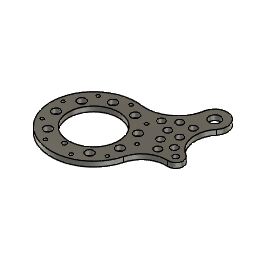
电机支架面板2 v8 (Autodesk Fusion 360 design; units mm, degrees)
Autodesk Fusion 360 part; units mm, degrees
sketch "草图1" plane through (0, 0, 0) normal (0, 0, 1) x (1, 0, 0)
  circle A0 centre (0, 0) radius 25
  circle A1 centre (0, 0) radius 37.5 construction
  circle A2 centre (0, 0) radius 42.5
  line L0 (0, 0) -> (0, 56.853) construction
  circle A3 centre (0, 37.5) radius 1.65
  circle A4 centre (-24.1045, 28.7267) radius 1.65
  circle A5 centre (-36.9303, 6.5118) radius 1.65
  circle A6 centre (-32.476, -18.75) radius 1.65
  circle A7 centre (-12.8258, -35.2385) radius 1.65
  circle A8 centre (12.8258, -35.2385) radius 1.65
  circle A9 centre (32.476, -18.75) radius 1.65
  circle A10 centre (36.9303, 6.5118) radius 1.65
  circle A11 centre (24.1045, 28.7267) radius 1.65
  line L1 (0, 0) -> (0, -49) construction
  circle A12 centre (0, -29) radius 2.2361
  dimension "d1" = 50
  dimension "d2" = 75
  dimension "d3" = 85
  dimension "d4" = 3.3
  dimension "d6" = 360
  dimension "d8" = 29
  constraint coincident A0.centre A1.centre
  constraint concentric A0 A1
  constraint concentric A0 A2
  constraint vertical L0
  constraint coincident A1 A3.centre
  constraint coincident L0 A3.centre
  constraint parallel L0 L1
  constraint coincident L1 A12.centre
  measures "d1" diameter of A0
  measures "d2" diameter of A1
  measures "d3" diameter of A2
  measures "d4" diameter of A3
  measures "d8" distance of A0.centre A12.centre
extrude "拉伸1" add sketch "草图1" along normal blind 5
sketch "草图3" plane through (0, 0, 0) normal (0, 0, 1) x (1, 0, 0)
  circle A0 centre (67, 15) radius 2.75
  circle A1 centre (54.28, 66.715) radius 5.5
  circle A2 centre (67, 15) radius 7.5
  circle A3 centre (54.28, 66.715) radius 12.5
  circle A4 centre (0, 0) radius 42.5
  line L0 (66.6449, 68.5478) -> (74.4189, 16.0997)
  line L1 (-68.0785, 9.2748) -> (71.3613, 91.2584)
  line L2 (-3.0488, -61.2363) -> (103.0722, 38.6545)
  circle A5 centre (65.2053, -17.4504) radius 25
  circle A6 centre (9.9306, 74.3396) radius 32.5
  circle A7 centre (83.3843, 43.0678) radius 25
  circle A8 centre (52.1934, 33.8453) radius 3.5
  circle A9 centre (58.5588, 22.0531) radius 3.5
  circle A10 centre (51.2685, 48.2157) radius 3.5
  circle A11 centre (40.298, 33.8483) radius 3.5
  circle A12 centre (44.4546, 22.4304) radius 3.5
  circle A13 centre (83.3843, 43.0678) radius 29.0258
  circle A14 centre (83.3843, 43.0678) radius 40.5617
  circle A15 centre (51.5586, 12.5957) radius 3.5
  circle A16 centre (39.4668, 46.6293) radius 3.5
  circle A17 centre (0, 0) radius 28.4164
  circle A18 centre (0, -32.4164) radius 4
  circle A19 centre (20.8369, -24.8324) radius 4
  circle A20 centre (31.9239, -5.629) radius 4
  circle A21 centre (28.0734, 16.2082) radius 4
  circle A22 centre (11.0871, 30.4614) radius 4
  circle A23 centre (-11.0871, 30.4614) radius 4
  circle A24 centre (-28.0734, 16.2082) radius 4
  circle A25 centre (-31.9239, -5.629) radius 4
  circle A26 centre (-20.8369, -24.8324) radius 4
  circle A27 centre (28.9963, 38.608) radius 3.5
  circle A28 centre (9.9306, 74.3396) radius 37
  circle A29 centre (65.2053, -17.4504) radius 29.5
  dimension "d11" = 5.5
  dimension "d12" = 11
  dimension "d15" = 15
  dimension "d16" = 25
  dimension "d18" = 85
  dimension "d21" = 51.715
  dimension "d22" = 12.72
  dimension "d30" = 67
  dimension "d31" = 15
  dimension "d32" = 50
  dimension "d33" = 65
  dimension "d34" = 50
  dimension "d35" = 7
  dimension "d36" = 7
  dimension "d37" = 7
  dimension "d38" = 7
  dimension "d40" = 7
  dimension "d41" = 4.0258
  dimension "d42" = 15.5617
  dimension "d43" = 7
  dimension "d44" = 7
  dimension "d45" = -14.0836
  dimension "d46" = 8
  dimension "d48" = 360
  dimension "d51" = 7
  dimension "d52" = 4.5
  dimension "d53" = 4.5
  constraint concentric A0 A2
  constraint concentric A1 A3
  constraint coincident A4.centre A17.centre
  constraint tangent A3 L0
  constraint tangent A2 L0
  constraint coincident A3 L0.start
  constraint coincident A2 L0.end
  constraint tangent A4 L1
  constraint tangent A3 L1
  constraint tangent A4 L2
  constraint tangent A2 L2
  constraint tangent A4 A5
  constraint tangent A2 A5
  constraint tangent A4 A6
  constraint tangent A3 A6
  constraint tangent A3 A7
  constraint tangent A2 A7
  constraint tangent A10 A13
  constraint tangent A8 A13
  constraint tangent A9 A13
  constraint tangent A11 A14
  constraint tangent A12 A14
  constraint tangent A2 A9
  constraint tangent A17 A18
  constraint vertical A4.centre A18.centre
  constraint tangent A27 A28
  constraint tangent A16 A28
  constraint tangent A15 A29
  constraint tangent A14 A15
  constraint tangent A14 A16
  measures "d11" diameter of A0
  measures "d12" diameter of A1
  measures "d15" diameter of A2
  measures "d16" diameter of A3
  measures "d18" diameter of A4
  measures "d21" vertical distance of A0.centre A1.centre
  measures "d22" horizontal distance of A0.centre A1.centre
  measures "d30" horizontal distance of A4.centre A0.centre
  measures "d31" vertical distance of A0.centre A4.centre
  measures "d32" diameter of A5
  measures "d33" diameter of A6
  measures "d34" diameter of A7
  measures "d35" diameter of A8
  measures "d36" diameter of A9
  measures "d37" diameter of A10
  measures "d38" diameter of A11
  measures "d40" diameter of A12
  measures "d43" diameter of A15
  measures "d44" diameter of A16
  measures "d46" diameter of A18
  measures "d51" diameter of A27
extrude "拉伸3" add sketch "草图3" along normal blind 5 contours A1 A3 A13 A14 | A1 A3 A14 A28 | A3 A14 A16 A28 | A2 A3 A9 A13 A14 A29 | A3 A4 A6 A28 | A3 A28 | A3 A13 | A2 A3 A7 A13 | A4 A14 A15 A16 A28 A29 | A2 A13 | A2 A29 | A2 A13 A29 | A2 A9 A13 | A14 A15 A29 | A2 A5 A14 A29 | A4 A5 A14 A29
extrude "拉伸4" cut sketch "草图3" along normal blind 11 contours A20 | A19 | A26 | A25 | A24 | A23 | A22 | A21
equation "d11 = 2.75 * 2 mm"
